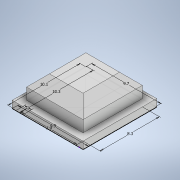
# Autodesk Inventor part: 1x led strip diffuser
Saved by Autodesk Inventor 2022 (Build 260153000, 153)
## iProperties
Created: 2022-04-12
Part Number: 1x led strip diffuser
Material: Generic
Document SubType Name: Modeling
Designer: a-dubs
Density: 1 g/cm^3
Appearance: Default
Author: a-dubs
Autodesk Inventor part; units mm, degrees
ref_plane "YZ Plane" through (0, 0, 0) normal (1, 0, 0) x (0, 1, 0)
ref_plane "XZ Plane" through (0, 0, 0) normal (0, 1, 0) x (-1, 0, 0)
ref_plane "XY Plane" through (0, 0, 0) normal (0, 0, 1) x (1, 0, 0)
sketch "Sketch1" plane through (0, 0, 0) normal (0, 1, 0) x (-1, 0, 0)
  line L0 (0, 0) -> (-9.9, 0)
  line L1 (0, 0) -> (0, -10.3)
  line L2 (0, -10.3) -> (-9.9, -10.3)
  line L3 (-9.9, -10.3) -> (-9.9, 0)
  line L4 (-9.9, -10.3) -> (-9.4, -10.3)
  line L5 (0, -10.3) -> (-0.5, -10.3)
  line L6 (-0.5, 0) -> (-1.5, 0)
  line L7 (-4.95, 0) -> (-4.95, -10.3)
  line L8 (-1, -9.3) -> (-8.9, -9.3)
  line L9 (-8.9, -9.3) -> (-8.9, -1)
  line L10 (-8.9, -1) -> (-1, -1)
  line L11 (-1, -1) -> (-1, -9.3)
  line L12 (-1, -9.3) -> (-8.9, -1) construction
  line L13 (-8.9, -9.3) -> (-1, -1) construction
  line L14 (-9.8, -0.1) -> (-0.1, -0.1)
  line L15 (-0.1, -0.1) -> (-0.1, -10.2)
  line L16 (-0.1, -10.2) -> (-9.8, -10.2)
  line L17 (-9.8, -10.2) -> (-9.8, -0.1)
  line L18 (-9.8, -0.1) -> (-0.1, -10.2) construction
  line L19 (-0.1, -0.1) -> (-9.8, -10.2) construction
  point P0 (-9.4, 0)
  point P1 (-4.95, -5.15)
  dimension "d0" = 9.9
  dimension "d1" = 10.3
  dimension "d40" = 1
  dimension "d41" = 7.9
  dimension "d42" = 8.3
  dimension "d50" = 9.7
  dimension "d51" = 10.1
  constraints: 40 end point, 7 midpoint, 5 point on line, 4 parallel, 4 perpendicular, 3 horizontal, 1 vertical
  measures "d0" distance of L0.start L0.end
  measures "d1" distance of L0.start L1.end
  measures "d40" distance of L6.start L6.end
  measures "d41" distance of L9.end L10.end
  measures "d42" distance of L8.end L9.end
  measures "d50" distance of L15.end L16.end
  measures "d51" distance of L14.end L15.end
extrude "Extrusion6" add sketch "Sketch1" along normal blind 1
extrude "Extrusion7" add sketch "Sketch1" along normal blind 3.2 from surface at 1 contours L10 L11 L8 L7 | L7 L8 L9 L10
chamfer "Chamfer2" distance 1.6 angle 45 4 edges at (1, 4.2, -5.15) (4.95, 4.2, -1) (8.9, 4.2, -5.15) (4.95, 4.2, -9.3)
body "Solid2"
